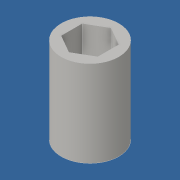
# Autodesk Inventor part: 8mm spacer
Saved by Autodesk Inventor 2016 (Build 200138000, 138)
## iProperties
Created: 2017-05-10
Part Number: 8mm spacer
Material: Generisch
Document SubType Name: Modeling
Designer: 4ndreas
Density: 1 g/cm^3
Appearance: Vorgabe
Author: 4ndreas
Autodesk Inventor part; units mm, degrees
ref_plane "YZ Plane" through (0, 0, 0) normal (1, 0, 0) x (0, 1, 0)
ref_plane "XZ Plane" through (0, 0, 0) normal (0, 1, 0) x (-1, 0, 0)
ref_plane "XY Plane" through (0, 0, 0) normal (0, 0, 1) x (1, 0, 0)
sketch "Skizze1" plane through (0, 0, 0) normal (0, 0, 1) x (1, 0, 0)
  circle A0 centre (0, 0) radius 4
  circle A1 centre (0, 0) radius 1.75
  dimension "d0" = 3.5
  dimension "d1" = 8
  constraints: 2 centre point, 2 coincident
  measures "d0" diameter of A1
  measures "d1" diameter of A0
extrude "Extrusion1" add sketch "Skizze1" along normal blind 12
sketch "Skizze2" plane through (0, 0, 12) normal (0, 0, 1) x (1, 0, 0)
  circle A0 centre (0, 0) radius 1.75 projected
  circle A1 centre (0, 0) radius 4 projected
  line L0 (0, 2.9445) -> (2.55, 1.4722)
  line L1 (2.55, 1.4722) -> (2.55, -1.4722)
  line L2 (2.55, -1.4722) -> (0, -2.9445)
  line L3 (0, -2.9445) -> (-2.55, -1.4722)
  line L4 (-2.55, -1.4722) -> (-2.55, 1.4722)
  line L5 (-2.55, 1.4722) -> (0, 2.9445)
  dimension "d4" = 5.1
  constraints: 12 end point, 1 coincident, 1 vertical, 13 other
  measures "d4" distance between parallel lines of L4 L1
extrude "Extrusion2" cut sketch "Skizze2" against normal blind 4 contours A0 | L0 L1 L2 L3 L4 L5
